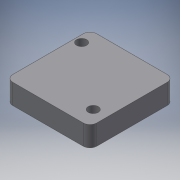
# Autodesk Inventor part: Hotend Lock 3
Saved by Autodesk Inventor 2016 SP1 (Build 200210100, 210)
## iProperties
Created: 2015-12-22
Part Number: Hotend Lock 3
Material: Generic
Document SubType Name: Modeling
Designer: PowerStation9000
Density: 1 g/cm^3
Appearance: Default
Author: PowerStation9000
Autodesk Inventor part; units mm, degrees
ref_plane "YZ Plane" through (0, 0, 0) normal (1, 0, 0) x (0, 1, 0)
ref_plane "XZ Plane" through (0, 0, 0) normal (0, 1, 0) x (-1, 0, 0)
ref_plane "XY Plane" through (0, 0, 0) normal (0, 0, 1) x (1, 0, 0)
sketch "Sketch1" plane through (0, 0, 0) normal (0, 0, 1) x (1, 0, 0)
  circle A0 centre (21, 6.9652) radius 1.5 construction
  circle A1 centre (21, 6.9652) radius 1.5 construction
  line L0 (25, 0) -> (16.5, 0) construction
  line L1 (25, 0) -> (25, 55) construction
  line L2 (0, 55) -> (25, 55) construction
  line L3 (0, 0) -> (0, 55) construction
  line L4 (0.5, 0) -> (0, 0) construction
  line L5 (0.5, 17) -> (16.5, 17) construction
  circle A2 centre (16, 45) radius 7.5 construction
  line L6 (2, 25) -> (23, 25)
  line L7 (25, 23) -> (25, 2)
  line L8 (23, 0) -> (2, 0)
  line L9 (0, 2) -> (0, 23)
  circle A3 centre (21, 6.9652) radius 1.5
  arc A4 (2, 25) -> (0, 23) centre (2, 23) ccw
  arc A5 (0, 2) -> (2, 0) centre (2, 2) ccw
  arc A6 (23, 0) -> (25, 2) centre (23, 2) ccw
  arc A7 (25, 23) -> (23, 25) centre (23, 23) ccw
  circle A8 centre (2, 20.5) radius 1.5
  circle A9 centre (2, 20.5) radius 1.5 projected
  line L10 (14.5, 12) -> (14.5, 6) projected
  line L11 (14.5, 6) -> (16.5, 6) projected
  line L12 (16.5, 6) -> (16.5, 0) projected
  line L13 (0.5, 0) -> (0.5, 6) projected
  line L14 (0.5, 6) -> (2.5, 6) projected
  line L15 (2.5, 6) -> (2.5, 12) projected
  line L16 (2.5, 12) -> (0.5, 12) projected
  line L17 (0.5, 12) -> (0.5, 17) projected
  line L18 (16.5, 17) -> (16.5, 12) projected
  line L19 (16.5, 12) -> (14.5, 12) projected
  point P0 (0, 25)
  dimension "d0" = 25
  dimension "d1" = 3
  dimension "d2" = 2
  dimension "d5" = 3
  dimension "d6" = 2
  dimension "d7" = 4.5
  constraints: 8 end point, 8 point on circle, 8 tangent, 6 centre point, 5 point on line, 3 equal radius, 2 parallel, 1 coincident, 1 horizontal, 1 perpendicular
  measures "d0" distance between parallel lines of L8 L6
  measures "d1" diameter of A3
  measures "d2" radius of A4
  measures "d5" diameter of A8
  measures "d6" distance from line of L9 A8.centre
  measures "d7" distance from line of L6 A8.centre
extrude "Extrusion1" add sketch "Sketch1" along normal blind 6
sketch "Sketch2" plane through (2, 0, 0) normal (0, -1, 0) x (1, 0, 0)
  circle A0 centre (6.5, -5) radius 8 construction
  circle A1 centre (6.5, -5) radius 8
  line L0 (21, 0) -> (0, 0) projected
  line L1 (0, 0) -> (0, 6) projected
  line L2 (21, 6) -> (0, 6) projected
  line L3 (21, 0) -> (21, 6) projected
  line L4 (12.745, 0) -> (0.255, 0)
  point P0 (-2, 0)
  constraints: 2 end point, 2 point on circle, 2 point on line, 1 centre point, 1 coincident, 1 concentric
extrude "Extrusion2" cut sketch "Sketch2" against normal blind 17 contours L0 A1 picked at (4.8404, 0.4206)
body "Solid1"
